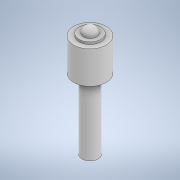
# Autodesk Inventor part: Rodillo_Sostener
Saved by Autodesk Inventor 2021 (Build 250183000, 183)
## iProperties
Created: 2021-06-07
Part Number: Rodillo_Sostener
Material: Genérico
Document SubType Name: Modeling
Designer: Mecatronica
Density: 1 g/cm^3
Appearance: Valor por defecto
Author: Mecatronica
Autodesk Inventor part; units mm, degrees
ref_plane "YZ Plane" through (0, 0, 0) normal (1, 0, 0) x (0, 1, 0)
ref_plane "XZ Plane" through (0, 0, 0) normal (0, 1, 0) x (-1, 0, 0)
sketch "Boceto1" plane through (0, 0, 0) normal (0, 1, 0) x (-1, 0, 0)
  circle A0 centre (0, 0) radius 15
  dimension "d0" = 30
  constraints: 1 centre point, 1 coincident
  measures "d0" diameter of A0
extrude "Extrusión1" add sketch "Boceto1" along normal blind 30
sketch "Boceto4" plane through (0, 30, 0) normal (0, 1, 0) x (1, 0, 0)
  circle A0 centre (0, 0) radius 10
  dimension "d7" = 20
  constraints: 1 centre point, 1 coincident
  measures "d7" diameter of A0
extrude "Extrusión2" add sketch "Boceto4" along normal blind 2
sketch "Boceto5" plane through (0, 32, 0) normal (0, 1, 0) x (1, 0, 0)
  circle A0 centre (0, 0) radius 10 projected
  line L0 (-10, 0) -> (10, 0)
  constraints: 2 end point, 2 point on circle, 1 horizontal
ref_plane "Plano de trabajo2" through (-10, 32, 0) normal (0, 0, 1) x (1, 0, 0)
sketch "Boceto6" plane through (-10, 32, 0) normal (0, 0, 1) x (1, 0, 0)
  line L0 (20, 0) -> (0, 0) projected
  circle A0 centre (10, 0) radius 6
  line L1 (4, 0) -> (16, 0)
  point P0 (10, -32)
  dimension "d11" = 12
  constraints: 2 end point, 2 point on circle, 1 centre point, 1 midpoint, 1 point on line
  measures "d11" diameter of A0
revolve "Revolución2" add sketch "Boceto6" angle 360 about axis through (-6, 32, 0) along (1, 0, 0) picked at (11.497, 2.2835) contours L0 A0
sketch "Boceto7" plane through (0, 0, 0) normal (0, -1, 0) x (1, 0, 0)
  circle A0 centre (0, 0) radius 7.5
  dimension "d13" = 15
  constraints: 1 centre point, 1 coincident
  measures "d13" diameter of A0
extrude "Extrusión3" add sketch "Boceto7" along normal blind 65
